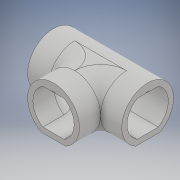
# Autodesk Inventor part: T corridor
Saved by Autodesk Inventor 2017 (Build 210142000, 142)
## iProperties
Created: 2018-03-04
Part Number: T corridor
Material: Generic
Document SubType Name: Modeling
Designer: Braxton
Density: 1 g/cm^3
Appearance: Default
Author: Braxton
Autodesk Inventor part; units mm, degrees
ref_plane "YZ Plane" through (0, 0, 0) normal (1, 0, 0) x (0, 1, 0)
ref_plane "XZ Plane" through (0, 0, 0) normal (0, 1, 0) x (-1, 0, 0)
sketch "Sketch1" plane through (0, 0, 0) normal (1, 0, 0) x (0, 1, 0)
  line L0 (-84.666667, 50.8) -> (-84.666667, -50.8)
  arc A0 (-110.066667, -57.405887) -> (-110.066667, 57.405887) centre (0, 0) ccw
  arc A1 (84.666667, 50.8) -> (-84.666667, 50.8) centre (0, 0) ccw
  arc A2 (-84.666667, -50.8) -> (84.666667, -50.8) centre (0, 0) ccw
  line L1 (-110.066667, -57.405887) -> (-110.066667, 57.405887)
  line L2 (84.666667, 8.995833) -> (84.666667, -8.995833) construction
  arc A3 (86.254167, -7.408333) -> (84.666667, -8.995833) centre (86.254167, -8.995833) ccw
  arc A4 (84.666667, 8.995833) -> (86.254167, 7.408333) centre (86.254167, 8.995833) ccw
  line L3 (87.841667, 7.408333) -> (86.254167, 7.408333)
  line L4 (87.841667, -7.408333) -> (86.254167, -7.408333)
  line L5 (87.841667, 7.408333) -> (87.841667, -7.408333)
  line L6 (84.666667, 0) -> (87.841667, 0) construction
  line L7 (84.666667, 50.8) -> (84.666667, 8.995833)
  line L8 (84.666667, -8.995833) -> (84.666667, -50.8)
  line L9 (84.646092, 4.084376) -> (84.646092, 0)
  line L10 (87.841667, 6.35) -> (87.841667, 0)
  line L11 (87.841667, 6.35) -> (86.892655, 6.35)
  line L12 (84.666733, 6.32944) -> (88.444674, 2.551499) construction
  arc A5 (86.892655, 6.35) -> (84.646092, 4.084376) centre (86.911797, 4.084376) ccw
  arc A6 (84.646092, 3.154507) -> (87.841667, 6.35) centre (84.666733, 6.32944) ccw construction
  line L13 (84.646092, 0) -> (87.841667, 0) construction
  line L14 (84.646092, -4.084376) -> (84.646092, 0)
  line L15 (87.841667, -6.35) -> (87.841667, 0)
  arc A7 (87.841667, -6.35) -> (84.646092, -3.154507) centre (84.666733, -6.32944) ccw construction
  arc A8 (84.646092, -4.084376) -> (86.892655, -6.35) centre (86.911797, -4.084376) ccw
  line L16 (84.666733, -6.32944) -> (88.444674, -2.551499) construction
  line L17 (87.841667, -6.35) -> (86.892655, -6.35)
  dimension "d1" = 101.6
  dimension "d2" = 248.2749
  dimension "d41" = 25.4
  dimension "d56" = 14.81667
  dimension "d57" = 1.5875
  dimension "d58" = 1.5875
  dimension "d65" = 6.35
  dimension "d66" = 3.175
  dimension "d67" = 45
  dimension "d68" = 2.26571
  dimension "d69" = 2.24656
  dimension "d110" = 84.66667
  constraints: 36 end point, 20 point on circle, 11 symmetric about line, 9 centre point, 4 coincident, 4 point on line, 3 vertical, 2 parallel, 2 perpendicular, 2 tangent, 1 midpoint, 3 other
  measures "d1" distance of L7.start L8.end
  measures "d2" diameter of A0
  measures "d41" distance between parallel lines of L0 L1
  measures "d56" distance of L3.start L4.start
  measures "d57" distance from line of L2.end L4
  measures "d58" radius of A3
  measures "d65" distance of L10.end L10.start
  measures "d66" distance of L10.start L12.start
  measures "d67" angle of L10 L12
  measures "d68" radius of A5
  measures "d69" horizontal distance of L9.start L11.end
  measures "d110" distance from line of L8 A0.centre
extrude "corridor" add sketch "Sketch1" against normal blind 101.6
extrude "light right of T" add sketch "Sketch1" against normal up to surface (101.6 mm away) separate body contours L5 L17 A8 L14 L9 A5 L11
ref_plane "Work Plane1" through (0, 0, -124.137452) normal (0, 0, 1) x (1, 0, 0)
sketch "Sketch4" plane through (0, 0, -124.137452) normal (0, 0, 1) x (1, 0, 0)
  line L0 (73.337452, -84.666667) -> (174.937452, -84.666667)
  arc A0 (181.543339, -110.066667) -> (66.731565, -110.066667) centre (124.137452, 0) ccw
  arc A1 (73.337452, 84.666667) -> (73.337452, -84.666667) centre (124.137452, 0) ccw
  arc A2 (174.937452, -84.666667) -> (174.937452, 84.666667) centre (124.137452, 0) ccw
  line L1 (0, -110.066667) -> (0, 124.137452)
  line L2 (181.543339, -110.066667) -> (66.731565, -110.066667)
  line L3 (124.137452, 84.666667) -> (124.137452, 87.841667) construction
  line L4 (116.729119, 87.841667) -> (116.729119, 86.254167)
  line L5 (131.545785, 87.841667) -> (131.545785, 86.254167)
  line L6 (115.141619, 84.666667) -> (133.133285, 84.666667) construction
  arc A3 (131.545785, 86.254167) -> (133.133285, 84.666667) centre (133.133285, 86.254167) ccw
  arc A4 (115.141619, 84.666667) -> (116.729119, 86.254167) centre (115.141619, 86.254167) ccw
  line L7 (73.337452, 84.666667) -> (115.141619, 84.666667)
  line L8 (133.133285, 84.666667) -> (174.937452, 84.666667)
  line L9 (117.787452, 87.841667) -> (117.787452, 86.617832)
  line L10 (120.034015, 84.646026) -> (124.137452, 84.646026)
  line L11 (124.137452, 84.646026) -> (124.137452, 87.841667) construction
  line L12 (117.788951, 84.666667) -> (120.963201, 87.840918) construction
  arc A5 (120.963884, 84.646026) -> (117.787452, 87.841667) centre (117.788951, 84.666667) ccw construction
  arc A6 (117.787452, 86.617832) -> (120.034015, 84.646026) centre (120.034015, 86.911731) ccw
  line L13 (130.487452, 87.841667) -> (130.487452, 86.617832)
  line L14 (128.240889, 84.646026) -> (124.137452, 84.646026)
  line L15 (130.485954, 84.666667) -> (127.311703, 87.840918) construction
  arc A7 (130.487452, 87.841667) -> (127.311021, 84.646026) centre (130.485954, 84.666667) ccw construction
  arc A8 (128.240889, 84.646026) -> (130.487452, 86.617832) centre (128.240889, 86.911731) ccw
  line L16 (131.545785, 87.841667) -> (130.487452, 87.841667)
  line L17 (130.487452, 87.841667) -> (124.137452, 87.841667)
  line L18 (124.137452, 87.841667) -> (117.787452, 87.841667)
  line L19 (117.787452, 87.841667) -> (116.729119, 87.841667)
  point P0 (0, 0)
  dimension "d7" = 101.6
  dimension "d8" = 248.2749
  dimension "d19" = 124.13745
  dimension "d42" = 25.4
  dimension "d88" = 14.81667
  dimension "d89" = 1.5875
  dimension "d90" = 1.5875
  dimension "d92" = 6.35
  dimension "d93" = 3.175
  dimension "d95" = 2.26571
  dimension "d96" = 2.24656
  constraints: 38 end point, 20 point on circle, 11 symmetric about line, 9 centre point, 4 coincident, 4 point on line, 3 collinear, 3 horizontal, 2 parallel, 2 perpendicular, 2 tangent, 2 vertical, 3 other
  measures "d7" distance of L7.start L8.end
  measures "d8" diameter of A0
  measures "d19" distance from line of L1 point (124.137, 0)
  measures "d42" distance between parallel lines of L0 L2
  measures "d88" distance of L4.start L5.start
  measures "d89" distance from line of L6.end L5
  measures "d90" radius of A3
  measures "d92" distance of L11.end L9.start
  measures "d93" distance of L9.start L12.start
  measures "d95" radius of A6
  measures "d96" horizontal distance of L10.start L9.end
extrude "T bottom" add sketch "Sketch4" against normal blind 101.6 bodies 1
extrude "light bottom of T" add sketch "Sketch4" against normal up to surface (101.6 mm away) separate body contours L18 L17 L13 A8 L14 L10 A6 L9
sketch "Sketch8" plane through (0, 0, 0) normal (1, 0, 0) x (0, 0, -1)
  arc A0 (124.137452, 0) -> (124.137452, 0) centre (0, 0) ccw
  line L0 (-8.995833, 84.666667) -> (-50.8, 84.666667)
  arc A1 (50.8, -84.666667) -> (50.8, 84.666667) centre (0, 0) ccw
  line L1 (50.8, -84.666667) -> (0, -84.666667)
  line L2 (-50.8, -84.666667) -> (50.8, -84.666667)
  line L3 (0, -84.666667) -> (0, -110.066667)
  arc A2 (124.137452, 0) -> (124.137452, 0) centre (0, 0) ccw
  arc A3 (50.8, -84.666667) -> (50.8, 84.666667) centre (0, 0) ccw
  arc A4 (57.405887, -110.066667) -> (0, 124.137452) centre (0, 0) ccw
  line L4 (57.405887, -110.066667) -> (-57.405887, -110.066667)
  line L5 (0, -110.066667) -> (57.405887, -110.066667)
  line L6 (0, 124.137452) -> (0, 87.841667)
  line L7 (7.408333, 87.841667) -> (-7.408333, 87.841667)
  line L8 (50.8, 84.666667) -> (8.995833, 84.666667)
  line L9 (50.8, 84.666667) -> (8.995833, 84.666667)
  arc A5 (7.408333, 86.254167) -> (8.995833, 84.666667) centre (8.995833, 86.254167) ccw
  arc A6 (7.408333, 86.254167) -> (8.995833, 84.666667) centre (8.995833, 86.254167) ccw
  line L10 (7.408333, 86.254167) -> (7.408333, 87.841667)
  line L11 (7.408333, 87.841667) -> (7.408333, 86.254167)
  line L12 (4.084376, 84.646092) -> (-4.084376, 84.646092)
  arc A7 (4.084376, 84.646092) -> (6.35, 86.892655) centre (4.084376, 86.911797) ccw
  line L13 (6.35, 87.841667) -> (6.35, 86.892655)
  arc A8 (4.084376, 84.646092) -> (6.35, 86.892655) centre (4.084376, 86.911797) ccw
  line L14 (-6.35, 87.841667) -> (6.35, 87.841667)
  line L15 (0, 87.841667) -> (6.35, 87.841667)
  line L16 (6.35, 87.841667) -> (7.408333, 87.841667)
  line L17 (6.35, 87.841667) -> (6.35, 86.892655)
  arc A9 (-6.35, 86.892655) -> (-4.084376, 84.646092) centre (-4.084376, 86.911797) ccw
  line L18 (-4.084376, 84.646092) -> (4.084376, 84.646092)
  line L19 (-6.35, 87.841667) -> (0, 87.841667)
  line L20 (-7.408333, 87.841667) -> (7.408333, 87.841667)
  line L21 (-6.35, 86.892655) -> (-6.35, 87.841667)
  line L22 (-6.35, 87.841667) -> (-6.35, 86.892655)
  arc A10 (-6.35, 86.892655) -> (-4.084376, 84.646092) centre (-4.084376, 86.911797) ccw
  point P0 (-29.897917, 84.666667)
  constraints: 24 end point, 10 point on circle, 7 collinear, 5 centre point, 4 midpoint, 3 tangent, 2 coincident, 2 vertical, 1 concentric, 1 point on line, 3 other
sketch "Sketch7" plane through (0, 0, 0) normal (0, 1, 0) x (-1, 0, 0)
  line L0 (0, -124.137452) -> (101.6, -124.137452)
  arc A0 (0, -98.737452) -> (-25.4, -124.137452) centre (0, -124.137452) ccw
  line L1 (-25.4, -124.137452) -> (-25.4, -225.737452) construction
  line L2 (0, -98.737452) -> (101.6, -98.737452) construction
  point P0 (0, 0)
  constraints: 4 end point, 3 point on circle, 2 point on line, 1 centre point, 1 tangent
sweep "corner curve" add profiles "Sketch8" path "Sketch7" bodies 1 path curves A0 contours A0 L4 L3 L1 A1 L8 A5 L10 L7 L6
sweep "light curve right" add profiles "Sketch8" path "Sketch7" separate body path curves A0 contours L7 L13 A7 L12 A9 L21
sketch "Sketch9" plane through (0, 0, 0) normal (1, 0, 0) x (0, 0, -1)
  line L0 (-6.35, 87.841667) -> (-7.408333, 87.841667)
  line L1 (-7.408333, 87.841667) -> (-7.408333, 86.254167)
  line L2 (-7.408333, 86.254167) -> (-7.408333, 87.841667)
  line L3 (-8.995833, 84.666667) -> (-50.8, 84.666667)
  line L4 (-8.995833, 84.666667) -> (-50.8, 84.666667)
  arc A0 (-8.995833, 84.666667) -> (-7.408333, 86.254167) centre (-8.995833, 86.254167) ccw
  arc A1 (-7.408333, 86.254167) -> (-7.408333, 86.254167) centre (-8.995833, 86.254167) ccw
  arc A2 (-8.995833, 84.666667) -> (-7.408333, 86.254167) centre (-8.995833, 86.254167) ccw
  line L5 (0, 87.841667) -> (0, 124.137452)
  arc A3 (57.405887, -110.066667) -> (-57.405887, -110.066667) centre (0, 0) ccw
  line L6 (-50.8, -84.666667) -> (50.8, -84.666667)
  line L7 (-50.8, -84.666667) -> (0, -84.666667)
  line L8 (0, -84.666667) -> (0, -110.066667)
  line L9 (57.405887, -110.066667) -> (-57.405887, -110.066667)
  line L10 (0, -110.066667) -> (-57.405887, -110.066667)
  arc A4 (0, 124.137452) -> (-57.405887, -110.066667) centre (0, 0) ccw
  arc A5 (-50.8, 84.666667) -> (-50.8, -84.666667) centre (0, 0) ccw
  arc A6 (-50.8, 84.666667) -> (-50.8, -84.666667) centre (0, 0) ccw
  line L11 (-6.35, 87.841667) -> (0, 87.841667)
  line L12 (6.35, 87.841667) -> (6.35, 86.892655)
  line L13 (0, 87.841667) -> (6.35, 87.841667)
  line L14 (6.35, 87.841667) -> (6.35, 86.892655)
  line L15 (4.084376, 84.646092) -> (-4.084376, 84.646092)
  line L16 (4.084376, 84.646092) -> (-4.084376, 84.646092)
  arc A7 (-6.35, 86.892655) -> (-4.084376, 84.646092) centre (-4.084376, 86.911797) ccw
  line L17 (-6.35, 86.892655) -> (-6.35, 87.841667)
  line L18 (-6.35, 87.841667) -> (-6.35, 86.892655)
  arc A8 (-6.35, 86.892655) -> (-4.084376, 84.646092) centre (-4.084376, 86.911797) ccw
  arc A9 (4.084376, 84.646092) -> (6.35, 86.892655) centre (4.084376, 86.911797) ccw
  arc A10 (4.084376, 84.646092) -> (6.35, 86.892655) centre (4.084376, 86.911797) ccw
  constraints: 24 end point, 11 point on circle, 6 collinear, 5 centre point, 5 concentric, 2 midpoint, 2 vertical, 1 horizontal alignment, 1 perpendicular, 1 tangent, 3 other
extrude "flat of T" add sketch "Sketch9" along normal blind 248.274904 contours L0 L1 A1 L3 A5 L6 L8 L9 A3 L5 L11 | A0 A1 bodies 1
extrude "light flat of T" add sketch "Sketch9" along normal up to surface (248.274904 mm away) separate body contours L11 L13 L12 A9 L15 A7 L17
sketch "Sketch10" plane through (248.274904, 0, 0) normal (1, 0, 0) x (0, 0, -1)
  line L0 (-50.8, -84.666667) -> (50.8, -84.666667)
  arc A0 (57.405887, -110.066667) -> (-57.405887, -110.066667) centre (0, 0) ccw
  arc A1 (-50.8, 84.666667) -> (-50.8, -84.666667) centre (0, 0) ccw
  arc A2 (50.8, -84.666667) -> (50.8, 84.666667) centre (0, 0) ccw
  line L1 (57.405887, -110.066667) -> (-57.405887, -110.066667)
  line L2 (-57.405887, -110.066667) -> (57.405887, -110.066667)
  arc A3 (-50.8, 84.666667) -> (-50.8, -84.666667) centre (0, 0) ccw
  line L3 (-8.995833, 84.666667) -> (-50.8, 84.666667)
  line L4 (-50.8, 84.666667) -> (-8.995833, 84.666667)
  line L5 (-7.408333, 87.841667) -> (-7.408333, 86.254167)
  line L6 (-7.408333, 86.254167) -> (-7.408333, 87.841667)
  line L7 (-6.35, 86.892655) -> (-6.35, 87.841667)
  line L8 (-7.408333, 87.841667) -> (-6.35, 87.841667)
  line L9 (6.35, 87.841667) -> (6.35, 86.892655)
  line L10 (-6.35, 87.841667) -> (6.35, 87.841667)
  line L11 (6.35, 87.841667) -> (6.35, 86.892655)
  line L12 (7.408333, 87.841667) -> (7.408333, 86.254167)
  line L13 (6.35, 87.841667) -> (7.408333, 87.841667)
  arc A4 (7.408333, 86.254167) -> (8.995833, 84.666667) centre (8.995833, 86.254167) ccw
  line L14 (7.408333, 87.841667) -> (7.408333, 86.254167)
  line L15 (8.995833, 84.666667) -> (50.8, 84.666667)
  line L16 (124.137452, 84.666667) -> (8.995833, 84.666667)
  arc A5 (-6.35, 86.892655) -> (-4.084376, 84.646092) centre (-4.084376, 86.911797) ccw
  arc A6 (4.084376, 84.646092) -> (6.35, 86.892655) centre (4.084376, 86.911797) ccw
  line L17 (4.084376, 84.646092) -> (-4.084376, 84.646092)
  line L18 (4.084376, 84.646092) -> (-4.084376, 84.646092)
  line L19 (-6.35, 86.892655) -> (-6.35, 87.841667)
  arc A7 (-8.995833, 84.666667) -> (-7.408333, 86.254167) centre (-8.995833, 86.254167) ccw
  arc A8 (-6.35, 86.892655) -> (-4.084376, 84.646092) centre (-4.084376, 86.911797) ccw
  arc A9 (4.084376, 84.646092) -> (6.35, 86.892655) centre (4.084376, 86.911797) ccw
  arc A10 (7.408333, 86.254167) -> (8.995833, 84.666667) centre (8.995833, 86.254167) ccw
  line L20 (124.137452, -110.066667) -> (225.737452, -110.066667)
  line L21 (124.137452, 124.137452) -> (124.137452, -110.066667) construction
  dimension "d25" = 101.6
  dimension "d26" = 248.2749
  constraints: 26 end point, 14 point on circle, 7 centre point, 7 collinear, 5 perpendicular, 5 tangent, 2 coincident, 1 concentric
  measures "d25" distance of L3.end L15.end
  measures "d26" diameter of A0
ref_plane "mirror plane" through (124.137452, 0, 0) normal (1, 0, 0) x (0, 0, 1)
extrude "other end of T" add sketch "Sketch10" along normal blind 101.6 bodies 1
extrude "other end of T light" add sketch "Sketch10" along normal up to surface (101.6 mm away) separate body contours L10 L9 A6 L17 A5 L7
mirror "corner curve mirror" about plane through (124.137452, 0, 0) normal (1, 0, 0) of "corner curve" bodies 1
revolve "light curve left" add sketch "Sketch10" angle 90 about axis through (248.274904, 124.137452, -124.137452) along (0, -1, 0) bodies 1 contours L10 L9 A6 L17 A5 L7
ref_plane "Work Plane3" through (0, 124.137452, 6.35) normal (0, 1, 0) x (1, 0, 0)
sketch "Sketch15" plane through (0, 124.137452, 6.35) normal (0, 1, 0) x (1, 0, 0)
  arc A0 (124.137452, 130.487452) -> (248.274904, 6.35) centre (248.274904, 130.487452) ccw
  arc A1 (124.137452, 130.487452) -> (248.274904, 6.35) centre (248.274904, 130.487452) ccw
  line L0 (0, 6.35) -> (248.274904, 6.35)
  arc A2 (0, 6.35) -> (124.137452, 130.487452) centre (0, 130.487452) ccw
  line L1 (0, 6.35) -> (248.274904, 6.35)
  constraints: 4 point on circle, 2 centre point, 2 end point, 1 concentric, 1 equal radius, 1 horizontal
extrude "top hole fill" add sketch "Sketch15" against normal up to surface (36.295785 mm away) bodies 5
sketch "Sketch16" plane through (39.194683, 87.841667, -6.35) normal (0, -1, 0) x (1, 0, 0)
  line L0 (-39.194683, 0) -> (209.080222, 0) construction
  line L1 (151.697356, 0) -> (18.188183, 0)
  line L2 (-39.194683, 2.265624) -> (209.080222, 2.265624)
  arc A0 (149.574004, -1.058333) -> (84.94277, -75.875996) centre (209.080222, -117.787452) ccw
  arc A1 (84.94277, -75.875996) -> (20.311535, -1.058333) centre (-39.194683, -117.787452) ccw
  line L3 (149.574004, -1.058333) -> (20.311535, -1.058333)
  point P0 (-39.194683, 6.35)
  point P1 (81.686564, -89.541546)
  dimension "d117" = 262.04333
  dimension "d118" = 262.04333
  dimension "d119" = 1.05833
  constraints: 4 end point, 4 point on circle, 2 centre point, 2 parallel
  measures "d117" diameter of A0
  measures "d118" diameter of A1
  measures "d119" distance between parallel lines of L3 L0
extrude "Extrusion18" add sketch "Sketch16" along normal blind 3.175 bodies 5
fillet "Fillet1" radius 1.5875 3 edges at (149.1252, 84.6667, -38.487) (99.1497, 84.6667, -38.487) (124.1375, 84.6667, -7.4083)
sketch "Sketch12" plane through (-101.6, -84.666667, 50.8) normal (0, 1, 0) x (1, 0, 0)
  arc A0 (101.6, 50.8) -> (225.737452, 174.937452) centre (101.6, 174.937452) ccw
  arc A1 (225.737452, 174.937452) -> (349.874904, 50.8) centre (349.874904, 174.937452) ccw
  line L0 (225.737452, 174.937452) -> (225.737452, 174.937452)
  line L1 (225.737452, 174.937452) -> (225.737452, 174.937452)
  line L2 (225.737452, 174.937452) -> (225.737452, 174.937452)
  line L3 (225.737452, 174.937452) -> (225.737452, 174.937452)
  line L4 (101.6, 50.8) -> (349.874904, 50.8)
  line L5 (101.6, 174.937452) -> (168.331565, 174.937452)
  arc A2 (101.6, 50.8) -> (225.737452, 174.937452) centre (101.6, 174.937452) ccw
  line L6 (283.143339, 174.937452) -> (349.874904, 174.937452)
  arc A3 (225.737452, 174.937452) -> (349.874904, 50.8) centre (349.874904, 174.937452) ccw
  constraints: 10 end point, 4 point on circle, 2 centre point, 2 concentric, 1 horizontal
equation "\"d57\" = 0.5 * d59"
equation "\"d22\" = d2"
equation "\"d5\" = -0.5 * d2"
equation "\"d59\" = 3.175"
body "Solid1"
body "Solid2"
body "Solid3"
body "Solid4"
body "Solid5"
body "Solid6"
